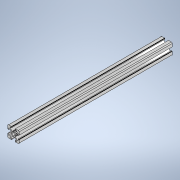
# Autodesk Inventor part: Profilés du réduit 20x20
Saved by Autodesk Inventor 2022 (Build 260153000, 153)
## iProperties
Created: 2021-12-06
Part Number: Profilés du réduit 20x20
Material: Générique
Document SubType Name: Modeling
Designer: utilisateur
Density: 1 g/cm^3
Appearance: Aluminum - Poli
Author: utilisateur
Autodesk Inventor part; units mm, degrees
ref_plane "YZ Plane" through (0, 0, 0) normal (1, 0, 0) x (0, 1, 0)
ref_plane "XZ Plane" through (0, 0, 0) normal (0, 1, 0) x (-1, 0, 0)
ref_plane "XY Plane" through (0, 0, 0) normal (0, 0, 1) x (1, 0, 0)
sketch "Esquisse1" plane through (0, 0, 0) normal (0, 0, 1) x (1, 0, 0)
  line L0 (-8.5, -10) -> (-3.5, -10)
  line L1 (-3.5, -10) -> (-3.5, -9.5)
  line L2 (-3.5, -9.5) -> (-3, -9.5)
  line L3 (-3, -9.5) -> (-3, -8.3)
  line L4 (-3, -8.3) -> (-5.2994, -8.3)
  arc A0 (-5.7944, -7.105) -> (-5.2994, -8.3) centre (-5.2994, -7.6) ccw
  line L5 (-5.7944, -7.105) -> (-2.1755, -3.4861)
  arc A1 (-1.6076, -3.388) -> (-2.1755, -3.4861) centre (-1.8219, -3.8397) ccw
  arc A2 (-1.6076, -3.388) -> (-0.3, -3.738) centre (0, 0) ccw
  line L6 (-0.3, -3.738) -> (0, -3.45)
  line L7 (0, -3.45) -> (0.3, -3.738)
  arc A3 (0.3, -3.738) -> (1.6076, -3.388) centre (0, 0) ccw
  arc A4 (2.1755, -3.4861) -> (1.6076, -3.388) centre (1.8219, -3.8397) ccw
  line L8 (2.1755, -3.4861) -> (5.7944, -7.105)
  arc A5 (5.2994, -8.3) -> (5.7944, -7.105) centre (5.2994, -7.6) ccw
  line L9 (5.2994, -8.3) -> (3, -8.3)
  line L10 (3, -8.3) -> (3, -9.5)
  line L11 (3, -9.5) -> (3.5, -9.5)
  line L12 (3.5, -9.5) -> (3.5, -10)
  line L13 (3.5, -10) -> (8.5, -10)
  arc A6 (8.5, -10) -> (10, -8.5) centre (8.5, -8.5) ccw
  line L14 (10, -8.5) -> (10, -3.5)
  line L15 (10, -3.5) -> (9.5, -3.5)
  line L16 (9.5, -3.5) -> (9.5, -3)
  line L17 (9.5, -3) -> (8.3, -3)
  line L18 (8.3, -3) -> (8.3, -5.2994)
  arc A7 (7.105, -5.7944) -> (8.3, -5.2994) centre (7.6, -5.2994) ccw
  line L19 (7.105, -5.7944) -> (3.4861, -2.1755)
  arc A8 (3.388, -1.6076) -> (3.4861, -2.1755) centre (3.8397, -1.8219) ccw
  arc A9 (3.388, -1.6076) -> (3.738, -0.3) centre (0, 0) ccw
  line L20 (3.738, -0.3) -> (3.45, 0)
  line L21 (3.45, 0) -> (3.738, 0.3)
  arc A10 (3.738, 0.3) -> (3.388, 1.6076) centre (0, 0) ccw
  arc A11 (3.4861, 2.1755) -> (3.388, 1.6076) centre (3.8397, 1.8219) ccw
  line L22 (3.4861, 2.1755) -> (7.105, 5.7944)
  arc A12 (8.3, 5.2994) -> (7.105, 5.7944) centre (7.6, 5.2994) ccw
  line L23 (8.3, 5.2994) -> (8.3, 3)
  line L24 (8.3, 3) -> (9.5, 3)
  line L25 (9.5, 3) -> (9.5, 3.5)
  line L26 (9.5, 3.5) -> (10, 3.5)
  line L27 (10, 3.5) -> (10, 8.5)
  arc A13 (10, 8.5) -> (8.5, 10) centre (8.5, 8.5) ccw
  line L28 (8.5, 10) -> (3.5, 10)
  line L29 (3.5, 10) -> (3.5, 9.5)
  line L30 (3.5, 9.5) -> (3, 9.5)
  line L31 (3, 9.5) -> (3, 8.3)
  line L32 (3, 8.3) -> (5.2994, 8.3)
  arc A14 (5.7944, 7.105) -> (5.2994, 8.3) centre (5.2994, 7.6) ccw
  line L33 (5.7944, 7.105) -> (2.1755, 3.4861)
  arc A15 (1.6076, 3.388) -> (2.1755, 3.4861) centre (1.8219, 3.8397) ccw
  arc A16 (1.6076, 3.388) -> (0.3, 3.738) centre (0, 0) ccw
  line L34 (0.3, 3.738) -> (0, 3.45)
  line L35 (0, 3.45) -> (-0.3, 3.738)
  arc A17 (-0.3, 3.738) -> (-1.6076, 3.388) centre (0, 0) ccw
  arc A18 (-2.1755, 3.4861) -> (-1.6076, 3.388) centre (-1.8219, 3.8397) ccw
  line L36 (-2.1755, 3.4861) -> (-5.7944, 7.105)
  arc A19 (-5.2994, 8.3) -> (-5.7944, 7.105) centre (-5.2994, 7.6) ccw
  line L37 (-5.2994, 8.3) -> (-3, 8.3)
  line L38 (-3, 8.3) -> (-3, 9.5)
  line L39 (-3, 9.5) -> (-3.5, 9.5)
  line L40 (-3.5, 9.5) -> (-3.5, 10)
  line L41 (-3.5, 10) -> (-8.5, 10)
  arc A20 (-8.5, 10) -> (-10, 8.5) centre (-8.5, 8.5) ccw
  line L42 (-10, 8.5) -> (-10, 3.5)
  line L43 (-10, 3.5) -> (-9.5, 3.5)
  line L44 (-9.5, 3.5) -> (-9.5, 3)
  line L45 (-9.5, 3) -> (-8.3, 3)
  line L46 (-8.3, 3) -> (-8.3, 5.2994)
  arc A21 (-7.105, 5.7944) -> (-8.3, 5.2994) centre (-7.6, 5.2994) ccw
  line L47 (-7.105, 5.7944) -> (-3.4861, 2.1755)
  arc A22 (-3.388, 1.6076) -> (-3.4861, 2.1755) centre (-3.8397, 1.8219) ccw
  arc A23 (-3.388, 1.6076) -> (-3.738, 0.3) centre (0, 0) ccw
  line L48 (-3.738, 0.3) -> (-3.45, 0)
  line L49 (-3.45, 0) -> (-3.738, -0.3)
  arc A24 (-3.738, -0.3) -> (-3.388, -1.6076) centre (0, 0) ccw
  arc A25 (-3.4861, -2.1755) -> (-3.388, -1.6076) centre (-3.8397, -1.8219) ccw
  line L50 (-3.4861, -2.1755) -> (-7.105, -5.7944)
  arc A26 (-8.3, -5.2994) -> (-7.105, -5.7944) centre (-7.6, -5.2994) ccw
  line L51 (-8.3, -5.2994) -> (-8.3, -3)
  line L52 (-8.3, -3) -> (-9.5, -3)
  line L53 (-9.5, -3) -> (-9.5, -3.5)
  line L54 (-9.5, -3.5) -> (-10, -3.5)
  line L55 (-10, -3.5) -> (-10, -8.5)
  arc A27 (-10, -8.5) -> (-8.5, -10) centre (-8.5, -8.5) ccw
  circle A28 centre (0, 0) radius 2.4
  dimension "d2" = 4.8
  constraints: 112 end point, 56 point on circle, 29 centre point, 20 horizontal, 20 vertical, 159 other
  measures "d2" diameter of A28
extrude "Extrusion1" add sketch "Esquisse1" along normal mid plane 268.3
